Autodesk Fusion 360 part; units mm, degrees
(part 3 of 5)
sketch "Sketch16" plane through (0, 0, 0) normal (0, -1, 0) x (-1, 0, 0)
  arc A0 (122.6742, -5.0956) -> (122.6212, -5.0863) centre (122.616, -5.2713) ccw
  line L0 (123.102, -5.144) -> (123.0752, -5.1645)
  line L1 (124.5216, -5.1639) -> (123.8644, -5.1286)
  arc A1 (123.6043, -5.242) -> (123.5882, -5.1255) centre (123.5845, -5.1854) ccw
  arc A2 (123.8233, -5.6545) -> (123.7767, -5.422) centre (122.7524, -5.7482) ccw
  arc A3 (123.856, -5.4349) -> (123.9598, -5.5039) centre (123.9512, -5.4043) ccw
  line L2 (123.789, -5.2264) -> (123.856, -5.4349)
  line L3 (123.3395, -5.8789) -> (123.7146, -5.8461)
  line L4 (123.7767, -5.422) -> (123.7544, -5.352)
  line L5 (121.8655, -5.4934) -> (125.5172, -5.6276)
  line L6 (123.8282, -5.7107) -> (123.8233, -5.6545)
  spline S0 degree 5 poles (122.9975, -5.9023) (123.1042, -5.893) (123.156, -5.8823) (123.1472, -5.7594) (123.0188, -5.7281) (122.9135, -5.8224) (122.9975, -5.9023) knots 0 0 0 0 0 0 0.5 1 1 1 1 1 1
  line L7 (122.9975, -5.9023) -> (123.1042, -5.893) construction
  line L8 (123.1042, -5.893) -> (123.156, -5.8823) construction
  line L9 (123.156, -5.8823) -> (123.1472, -5.7594) construction
  line L10 (123.1472, -5.7594) -> (123.0188, -5.7281) construction
  line L11 (123.0188, -5.7281) -> (122.9135, -5.8224) construction
  line L12 (122.9135, -5.8224) -> (122.9975, -5.9023) construction
  arc A4 (123.0752, -5.1645) -> (123.1045, -5.339) centre (123.1359, -5.244) ccw
  arc A5 (123.7146, -5.8461) -> (123.8282, -5.7107) centre (123.7037, -5.7216) ccw
  line L13 (123.1447, -5.7836) -> (123.2791, -5.8649)
  spline S1 degree 5 poles (122.9292, -5.3527) (122.88, -5.3469) (122.8215, -5.3033) (122.8246, -5.224) (122.8952, -5.1732) (122.9827, -5.2223) (122.9881, -5.3313) (122.9292, -5.3527) knots 0 0 0 0 0 0 0.333333 0.666667 1 1 1 1 1 1
  line L14 (122.9292, -5.3527) -> (122.88, -5.3469) construction
  line L15 (122.88, -5.3469) -> (122.8215, -5.3033) construction
  line L16 (122.8215, -5.3033) -> (122.8246, -5.224) construction
  line L17 (122.8246, -5.224) -> (122.8952, -5.1732) construction
  line L18 (122.8952, -5.1732) -> (122.9827, -5.2223) construction
  line L19 (122.9827, -5.2223) -> (122.9881, -5.3313) construction
  line L20 (122.9881, -5.3313) -> (122.9292, -5.3527) construction
  arc A6 (122.3543, -5.2288) -> (122.4452, -5.3073) centre (122.4233, -5.2408) ccw
  spline S2 degree 5 poles (122.4306, -5.4713) (122.4226, -5.3565) (122.5709, -5.3131) (122.7774, -5.2403) (122.8192, -5.3704) (122.8155, -5.4904) (122.7473, -5.545) (122.638, -5.5931) (122.5038, -5.5663) (122.4306, -5.4713) knots 0 0 0 0 0 0 0.2 0.4 0.6 0.8 1 1 1 1 1 1
  line L21 (122.4306, -5.4713) -> (122.4226, -5.3565) construction
  line L22 (122.4226, -5.3565) -> (122.5709, -5.3131) construction
  line L23 (122.5709, -5.3131) -> (122.7774, -5.2403) construction
  line L24 (122.7774, -5.2403) -> (122.8192, -5.3704) construction
  line L25 (122.8192, -5.3704) -> (122.8155, -5.4904) construction
  line L26 (122.8155, -5.4904) -> (122.7473, -5.545) construction
  line L27 (122.7473, -5.545) -> (122.638, -5.5931) construction
  line L28 (122.638, -5.5931) -> (122.5038, -5.5663) construction
  line L29 (122.5038, -5.5663) -> (122.4306, -5.4713) construction
  line L30 (122.6144, -5.6431) -> (122.606, -5.6464)
  line L31 (122.5301, -5.7335) -> (122.5128, -5.8052)
  arc A7 (122.8103, -5.6413) -> (122.6144, -5.6431) centre (122.7147, -5.8992) ccw
  line L32 (123.6245, -5.2886) -> (123.351, -5.3896)
  line L33 (123.1045, -5.339) -> (123.1299, -5.3473)
  arc A8 (124.6146, -5.2458) -> (124.5216, -5.1639) centre (124.5163, -5.2637) ccw
  line L34 (124.861, -5.7338) -> (124.2595, -5.7864)
  line L35 (123.3066, -5.3458) -> (123.6043, -5.242)
  arc A9 (123.7544, -5.352) -> (123.6245, -5.2886) centre (123.6591, -5.3824) ccw
  line L36 (121.8838, -4.9975) -> (125.5316, -5.1315)
  arc A10 (123.8644, -5.1286) -> (123.789, -5.2264) centre (123.8604, -5.2035) ccw
  line L37 (123.5882, -5.1255) -> (123.2358, -5.1035)
  line L38 (125.5137, -5.7485) -> (121.8444, -6.0696)
  line L39 (123.9598, -5.5039) -> (124.5079, -5.4565)
  spline S3 degree 5 poles (123.9494, -5.8171) (123.8625, -5.7888) (123.8706, -5.5918) (123.9121, -5.5354) (124.1515, -5.4258) (124.1212, -5.8274) (123.9494, -5.8171) knots 0 0 0 0 0 0 0.5 1 1 1 1 1 1
  line L40 (123.9494, -5.8171) -> (123.8625, -5.7888) construction
  line L41 (123.8625, -5.7888) -> (123.8706, -5.5918) construction
  line L42 (123.8706, -5.5918) -> (123.9121, -5.5354) construction
  line L43 (123.9121, -5.5354) -> (124.1515, -5.4258) construction
  line L44 (124.1515, -5.4258) -> (124.1212, -5.8274) construction
  line L45 (124.1212, -5.8274) -> (123.9494, -5.8171) construction
  line L46 (122.6795, -5.0974) -> (122.6742, -5.0956)
  arc A11 (122.8042, -5.9191) -> (122.8961, -5.8717) centre (122.798, -5.7943) ccw
  line L47 (122.3617, -5.1862) -> (122.3543, -5.2288)
  arc A12 (122.5128, -5.8052) -> (122.615, -5.9286) centre (122.61, -5.8287) ccw
  arc A13 (122.9027, -5.8633) -> (122.9181, -5.7333) centre (122.8047, -5.7858) ccw
  arc A14 (122.606, -5.6464) -> (122.5301, -5.7335) centre (122.6516, -5.7628) ccw
  spline S4 degree 5 poles (122.0426, -5.9763) (121.8729, -5.8903) (122.0398, -5.5137) (122.2556, -5.9869) (122.144, -6.0042) (122.0426, -5.9763) knots 0 0 0 0 0 0 1 1 1 1 1 1
  line L48 (122.0426, -5.9763) -> (121.8729, -5.8903) construction
  line L49 (121.8729, -5.8903) -> (122.0398, -5.5137) construction
  line L50 (122.0398, -5.5137) -> (122.2556, -5.9869) construction
  line L51 (122.2556, -5.9869) -> (122.144, -6.0042) construction
  line L52 (122.144, -6.0042) -> (122.0426, -5.9763) construction
  line L53 (122.8961, -5.8717) -> (122.9027, -5.8633)
  line L54 (122.615, -5.9286) -> (122.8042, -5.9191)
  line L55 (122.4452, -5.3073) -> (122.6793, -5.2304)
  arc A15 (122.9194, -5.7361) -> (122.8213, -5.6454) centre (122.7605, -5.8095) ccw
  line L56 (122.6212, -5.0863) -> (122.4884, -5.0826)
  line L57 (124.7695, -5.5577) -> (124.8858, -5.6544)
  line L58 (124.6105, -5.223) -> (124.6146, -5.2458)
  arc A16 (125.0173, -5.6732) -> (125.1878, -5.7213) centre (125.166, -5.4723) ccw
  line L59 (124.8259, -5.5315) -> (125.0173, -5.6732)
  spline S5 degree 5 poles (123.0947, -5.5531) (123.1905, -5.4657) (123.1798, -5.3896) (123.0478, -5.3646) (122.9193, -5.4022) (122.7897, -5.5433) (122.8659, -5.6259) (122.9658, -5.6557) (123.0537, -5.6399) (123.0947, -5.5531) knots 0 0 0 0 0 0 0.2 0.4 0.6 0.8 1 1 1 1 1 1
  line L60 (123.0947, -5.5531) -> (123.1905, -5.4657) construction
  line L61 (123.1905, -5.4657) -> (123.1798, -5.3896) construction
  line L62 (123.1798, -5.3896) -> (123.0478, -5.3646) construction
  line L63 (123.0478, -5.3646) -> (122.9193, -5.4022) construction
  line L64 (122.9193, -5.4022) -> (122.7897, -5.5433) construction
  line L65 (122.7897, -5.5433) -> (122.8659, -5.6259) construction
  line L66 (122.8659, -5.6259) -> (122.9658, -5.6557) construction
  line L67 (122.9658, -5.6557) -> (123.0537, -5.6399) construction
  line L68 (123.0537, -5.6399) -> (123.0947, -5.5531) construction
  arc A17 (125.4261, -5.2886) -> (125.3296, -5.1836) centre (125.3262, -5.2835) ccw
  arc A18 (123.116, -5.6386) -> (123.1447, -5.7836) centre (123.1964, -5.6981) ccw
  line L69 (125.3296, -5.1836) -> (124.7854, -5.1648)
  line L70 (123.2366, -5.4755) -> (123.116, -5.6386)
  arc A19 (124.861, -5.7338) -> (124.8858, -5.6544) centre (124.8571, -5.689) ccw
  arc A20 (123.351, -5.3896) -> (123.2366, -5.4755) centre (123.4377, -5.6241) ccw
  arc A21 (124.1566, -5.7201) -> (124.2595, -5.7864) centre (124.2508, -5.6868) ccw
  arc A22 (123.2791, -5.8649) -> (123.3395, -5.8789) centre (123.3308, -5.7793) ccw
  line L71 (124.1498, -5.6486) -> (124.1499, -5.6497)
  arc A23 (123.2358, -5.1035) -> (123.102, -5.144) centre (123.2233, -5.3031) ccw
  line L72 (125.5316, -5.1315) -> (125.5137, -5.7485)
  arc A24 (124.2379, -5.5417) -> (124.1499, -5.6497) centre (124.2495, -5.641) ccw
  line L73 (125.4094, -5.6154) -> (125.4261, -5.2886)
  arc A25 (123.1299, -5.3473) -> (123.3066, -5.3458) centre (123.2161, -5.0862) ccw
  line L74 (125.1878, -5.7213) -> (125.3183, -5.7099)
  arc A26 (125.3183, -5.7099) -> (125.4094, -5.6154) centre (125.3096, -5.6103) ccw
  line L75 (124.1566, -5.7201) -> (124.1559, -5.7183)
  arc A27 (124.6914, -5.3208) -> (124.8259, -5.5315) centre (125.0342, -5.2502) ccw
  line L76 (124.2379, -5.5417) -> (124.5806, -5.5016)
  line L77 (124.684, -5.2849) -> (124.6914, -5.3208)
  arc A28 (124.7854, -5.1648) -> (124.684, -5.2849) centre (124.7819, -5.2647) ccw
  arc A29 (124.7695, -5.5577) -> (124.5806, -5.5016) centre (124.6097, -5.7499) ccw
  line L78 (124.6271, -5.3138) -> (124.6105, -5.223)
  line L79 (124.1559, -5.7183) -> (124.1498, -5.6486)
  arc A30 (124.5079, -5.4565) -> (124.6136, -5.3988) centre (124.495, -5.3071) ccw
  arc A31 (124.6136, -5.3988) -> (124.6271, -5.3138) centre (124.4992, -5.3372) ccw
  line L80 (122.8213, -5.6454) -> (122.8103, -5.6413)
  line L81 (121.8444, -6.0696) -> (121.8838, -4.9975)
  spline S6 degree 5 poles (122.2381, -5.4004) (122.0382, -5.4442) (121.8814, -5.4184) (122.1972, -5.96) (122.3884, -6.05) (122.4454, -5.8928) (122.5168, -5.7223) (122.3409, -5.3698) (122.2381, -5.4004) knots 0 0 0 0 0 0 0.25 0.5 0.75 1 1 1 1 1 1
  line L82 (122.2381, -5.4004) -> (122.0382, -5.4442) construction
  line L83 (122.0382, -5.4442) -> (121.8814, -5.4184) construction
  line L84 (121.8814, -5.4184) -> (122.1972, -5.96) construction
  line L85 (122.1972, -5.96) -> (122.3884, -6.05) construction
  line L86 (122.3884, -6.05) -> (122.4454, -5.8928) construction
  line L87 (122.4454, -5.8928) -> (122.5168, -5.7223) construction
  line L88 (122.5168, -5.7223) -> (122.3409, -5.3698) construction
  line L89 (122.3409, -5.3698) -> (122.2381, -5.4004) construction
  arc A32 (122.6793, -5.2304) -> (122.6795, -5.0974) centre (122.6575, -5.1639) ccw
  arc A33 (122.1383, -5.3484) -> (122.2847, -5.1559) centre (122.0847, -5.1557) ccw
  line L90 (122.2098, -5.0785) -> (122.1123, -5.0784)
  line L91 (122.0124, -5.1715) -> (122.0048, -5.2817)
  line L92 (122.2847, -5.1559) -> (122.2847, -5.1536)
  arc A34 (122.4884, -5.0826) -> (122.3617, -5.1862) centre (122.4849, -5.2076) ccw
  arc A35 (122.0048, -5.2817) -> (122.0998, -5.3591) centre (122.0797, -5.2869) ccw
  arc A36 (122.2847, -5.1536) -> (122.2098, -5.0785) centre (122.2097, -5.1535) ccw
  arc A37 (122.1123, -5.0784) -> (122.0124, -5.1715) centre (122.1122, -5.1784) ccw
  line L93 (122.9181, -5.7333) -> (122.9194, -5.7361)
  line L94 (122.0998, -5.3591) -> (122.1383, -5.3484)
  arc A38 (101.6624, -9.2829) -> (105.8159, -15.1808) centre (107.6246, -9.4955) ccw
  arc A39 (70.9904, -13.8268) -> (76.2587, -14.0644) centre (73.9745, -6.1856) ccw
  arc A40 (89.9571, -7.1067) -> (89.8164, -11.0703) centre (90.5403, -9.1117) ccw
  line L95 (91.7075, -6.8404) -> (95.6704, -6.8748)
  arc A41 (109.7609, -10.0454) -> (106.8858, -7.1606) centre (106.7795, -10.1417) ccw
  arc A42 (99.3328, -10.1021) -> (95.6704, -6.8748) centre (95.6379, -10.6034) ccw
  line L96 (43.0155, -18.6474) -> (32.8431, -17.0766)
  line L97 (45.2455, -24.0556) -> (45.2666, -24.0022)
  line L98 (34.971, -7.0748) -> (54.6013, -6.7408)
  arc A43 (106.9529, -15.5425) -> (109.8673, -13.3383) centre (107.6312, -13.4105) ccw
  line L99 (45.5246, -21.9308) -> (45.5205, -21.9641)
  spline S7 degree 5 poles (96.9668, -18.5257) (97.3315, -15.1102) (92.9589, -13.6548) (86.882, -11.2585) (85.4937, -15.0929) (85.4728, -18.6727) (87.4465, -20.3757) (90.6533, -21.9288) (94.6811, -21.2769) (96.9668, -18.5257) knots 0 0 0 0 0 0 0.2 0.4 0.6 0.8 1 1 1 1 1 1
  line L100 (96.9668, -18.5257) -> (97.3315, -15.1102) construction
  line L101 (97.3315, -15.1102) -> (92.9589, -13.6548) construction
  line L102 (92.9589, -13.6548) -> (86.882, -11.2585) construction
  line L103 (86.882, -11.2585) -> (85.4937, -15.0929) construction
  line L104 (85.4937, -15.0929) -> (85.4728, -18.6727) construction
  line L105 (85.4728, -18.6727) -> (87.4465, -20.3757) construction
  line L106 (87.4465, -20.3757) -> (90.6533, -21.9288) construction
  line L107 (90.6533, -21.9288) -> (94.6811, -21.2769) construction
  line L108 (94.6811, -21.2769) -> (96.9668, -18.5257) construction
  line L109 (90.9724, -31.9544) -> (85.3412, -31.4649)
  line L110 (109.7609, -10.0454) -> (109.8673, -13.3383)
  line L111 (55.0443, -24.1326) -> (55.2523, -22.4622)
  arc A44 (91.3008, -23.4448) -> (85.4647, -23.1768) centre (88.0311, -30.9683) ccw
  arc A45 (56.7428, -9.7399) -> (54.6013, -6.7408) centre (54.6394, -8.9777) ccw
  arc A46 (91.7075, -6.8404) -> (90.1182, -7.0598) centre (91.6595, -12.3587) ccw
  line L112 (106.9529, -15.5425) -> (105.8159, -15.1808)
  line L113 (96.7132, -13.6191) -> (89.8164, -11.0703)
  spline S8 degree 5 poles (51.3155, -27.1729) (53.937, -26.4249) (53.9111, -20.5433) (52.7356, -18.8166) (45.7166, -15.2876) (46.1809, -27.2918) (51.3155, -27.1729) knots 0 0 0 0 0 0 0.5 1 1 1 1 1 1
  line L114 (51.3155, -27.1729) -> (53.937, -26.4249) construction
  line L115 (53.937, -26.4249) -> (53.9111, -20.5433) construction
  line L116 (53.9111, -20.5433) -> (52.7356, -18.8166) construction
  line L117 (52.7356, -18.8166) -> (45.7166, -15.2876) construction
  line L118 (45.7166, -15.2876) -> (46.1809, -27.2918) construction
  line L119 (46.1809, -27.2918) -> (51.3155, -27.1729) construction
  line L120 (101.6624, -9.2829) -> (101.6649, -9.2131)
  arc A47 (56.8948, -15.5841) -> (55.2523, -22.4622) centre (87.0737, -26.4258) ccw
  line L121 (69.427, -29.6816) -> (58.2835, -28.2936)
  line L122 (89.9571, -7.1067) -> (90.1182, -7.0598)
  arc A48 (55.0443, -24.1326) -> (58.2835, -28.2936) centre (58.7444, -24.5935) ccw
  arc A49 (96.7132, -13.6191) -> (99.5062, -11.3798) centre (97.4371, -11.6605) ccw
  line L123 (103.9805, -7.057) -> (106.8858, -7.1606)
  line L124 (99.3328, -10.1021) -> (99.5062, -11.3798)
  line L125 (75.3395, -27.0549) -> (71.244, -29.3293)
  arc A50 (62.837, -6.95) -> (62.232, -10.4064) centre (62.8831, -8.7392) ccw
  arc A51 (42.1027, -25.919) -> (45.2455, -24.0556) centre (42.4714, -22.9589) ccw
  line L126 (51.3477, -17.8246) -> (35.0606, -15.8132)
  arc A52 (103.9805, -7.057) -> (101.6649, -9.2131) centre (103.9007, -9.2928) ccw
  line L127 (113.7873, -4.9975) -> (4.8993, -5.006)
  arc A53 (72.9355, -17.7672) -> (69.6198, -15.0822) centre (66.7806, -21.9782) ccw
  line L128 (4.7576, -23.4188) -> (113.7898, -36.9995)
  line L129 (113.7884, -19.7997) -> (4.7873, -13.6679)
  line L130 (62.837, -6.95) -> (73.3676, -6.6788)
  line L131 (61.5787, -11.7716) -> (69.6198, -15.0822)
  line L132 (4.8993, -5.006) -> (4.7576, -23.4188)
  arc A54 (25.4984, -17.7008) -> (29.7394, -11.5664) centre (19.5973, -9.0879) ccw
  arc A55 (32.8431, -17.0766) -> (27.15, -18.542) centre (31.7051, -24.4468) ccw
  line L133 (32.258, -8.7389) -> (32.1089, -9.414)
  arc A56 (8.012, -19.5628) -> (10.626, -22.4806) centre (10.9947, -19.5204) ccw
  line L134 (25.4984, -17.7008) -> (19.6392, -21.7151)
  arc A57 (14.5024, -22.9634) -> (19.6392, -21.7151) centre (15.4242, -15.5631) ccw
  line L135 (56.8948, -15.5841) -> (57.6358, -13.5215)
  line L136 (14.5024, -22.9634) -> (10.626, -22.4806)
  line L137 (70.9904, -13.8268) -> (62.232, -10.4064)
  line L138 (24.2313, -23.693) -> (42.1027, -25.919)
  arc A58 (29.9989, -10.5044) -> (27.1075, -6.8132) centre (27.1011, -9.7962) ccw
  arc A59 (10.8624, -6.7785) -> (7.8733, -9.8039) centre (10.856, -9.7615) ccw
  line L139 (27.15, -18.542) -> (23.5773, -21.2981)
  arc A60 (31.6639, -11.4287) -> (31.9714, -13.9779) centre (35.4505, -12.2651) ccw
  line L140 (91.3008, -23.4448) -> (91.548, -23.5522)
  arc A61 (31.9714, -13.9779) -> (35.0606, -15.8132) centre (35.609, -11.3724) ccw
  arc A62 (23.5773, -21.2981) -> (24.2313, -23.693) centre (24.3972, -22.361) ccw
  line L141 (10.8624, -6.7785) -> (27.1075, -6.8132)
  line L142 (8.012, -19.5628) -> (7.8733, -9.8039)
  arc A63 (34.971, -7.0748) -> (32.1089, -9.414) centre (35.0217, -10.0574) ccw
  line L143 (72.9355, -17.7672) -> (76.3532, -22.7627)
  line L144 (31.6639, -11.4287) -> (32.258, -8.7389)
  line L145 (113.7898, -36.9995) -> (113.7873, -4.9975)
  line L146 (45.2666, -24.0022) -> (45.5246, -21.9308)
  line L147 (29.9989, -10.5044) -> (29.7394, -11.5664)
  line L148 (56.7428, -9.7399) -> (54.5179, -15.8803)
  spline S9 degree 5 poles (107.9837, -34.0023) (113.1348, -31.6237) (108.5717, -20.2166) (101.6226, -34.085) (104.9302, -34.7228) (107.9837, -34.0023) knots 0 0 0 0 0 0 1 1 1 1 1 1
  line L149 (107.9837, -34.0023) -> (113.1348, -31.6237) construction
  line L150 (113.1348, -31.6237) -> (108.5717, -20.2166) construction
  line L151 (108.5717, -20.2166) -> (101.6226, -34.085) construction
  line L152 (101.6226, -34.085) -> (104.9302, -34.7228) construction
  line L153 (104.9302, -34.7228) -> (107.9837, -34.0023) construction
  spline S10 degree 5 poles (77.0809, -20.2383) (74.3221, -17.5267) (74.7247, -15.2695) (78.6853, -14.6699) (82.4748, -15.9313) (86.1835, -20.2791) (83.823, -22.6567) (80.8115, -23.4352) (78.2106, -22.8684) (77.0809, -20.2383) knots 0 0 0 0 0 0 0.2 0.4 0.6 0.8 1 1 1 1 1 1
  line L154 (77.0809, -20.2383) -> (74.3221, -17.5267) construction
  line L155 (74.3221, -17.5267) -> (74.7247, -15.2695) construction
  line L156 (74.7247, -15.2695) -> (78.6853, -14.6699) construction
  line L157 (78.6853, -14.6699) -> (82.4748, -15.9313) construction
  line L158 (82.4748, -15.9313) -> (86.1835, -20.2791) construction
  line L159 (86.1835, -20.2791) -> (83.823, -22.6567) construction
  line L160 (83.823, -22.6567) -> (80.8115, -23.4352) construction
  line L161 (80.8115, -23.4352) -> (78.2106, -22.8684) construction
  line L162 (78.2106, -22.8684) -> (77.0809, -20.2383) construction
  spline S11 degree 5 poles (102.7832, -16.62) (108.6944, -18.1458) (113.3986, -17.5474) (103.3913, -33.3483) (97.5924, -35.8202) (96.0663, -31.0721) (94.1248, -25.9135) (99.7525, -15.5964) (102.7832, -16.62) knots 0 0 0 0 0 0 0.25 0.5 0.75 1 1 1 1 1 1
  line L163 (102.7832, -16.62) -> (108.6944, -18.1458) construction
  line L164 (108.6944, -18.1458) -> (113.3986, -17.5474) construction
  line L165 (113.3986, -17.5474) -> (103.3913, -33.3483) construction
  line L166 (103.3913, -33.3483) -> (97.5924, -35.8202) construction
  line L167 (97.5924, -35.8202) -> (96.0663, -31.0721) construction
  line L168 (96.0663, -31.0721) -> (94.1248, -25.9135) construction
  line L169 (94.1248, -25.9135) -> (99.7525, -15.5964) construction
  line L170 (99.7525, -15.5964) -> (102.7832, -16.62) construction
  arc A64 (77.31, -8.0343) -> (73.3676, -6.6788) centre (73.5212, -12.6428) ccw
  arc A65 (61.5787, -11.7716) -> (57.6358, -13.5215) centre (60.4431, -14.53) ccw
  arc A66 (45.5205, -21.9641) -> (43.0155, -18.6474) centre (42.5603, -21.5954) ccw
  line L171 (77.0236, -13.8427) -> (76.2587, -14.0644)
  line L172 (85.13, -23.287) -> (85.4647, -23.1768)
  spline S12 degree 5 poles (82.235, -14.4442) (83.7072, -14.324) (85.5003, -13.0901) (85.4918, -10.721) (83.4434, -9.1301) (80.7835, -10.4989) (80.5009, -13.7424) (82.235, -14.4442) knots 0 0 0 0 0 0 0.333333 0.666667 1 1 1 1 1 1
  line L173 (82.235, -14.4442) -> (83.7072, -14.324) construction
  line L174 (83.7072, -14.324) -> (85.5003, -13.0901) construction
  line L175 (85.5003, -13.0901) -> (85.4918, -10.721) construction
  line L176 (85.4918, -10.721) -> (83.4434, -9.1301) construction
  line L177 (83.4434, -9.1301) -> (80.7835, -10.4989) construction
  line L178 (80.7835, -10.4989) -> (80.5009, -13.7424) construction
  line L179 (80.5009, -13.7424) -> (82.235, -14.4442) construction
  line L180 (77.31, -8.0343) -> (78.0873, -8.6734)
  arc A67 (90.9724, -31.9544) -> (94.1541, -28.3895) centre (91.2307, -28.9826) ccw
  spline S13 degree 5 poles (79.5966, -30.7522) (76.4277, -30.3575) (74.8955, -29.9845) (75.29, -26.3298) (79.1534, -25.536) (82.1888, -28.4642) (79.5966, -30.7522) knots 0 0 0 0 0 0 0.5 1 1 1 1 1 1
  line L181 (79.5966, -30.7522) -> (76.4277, -30.3575) construction
  line L182 (76.4277, -30.3575) -> (74.8955, -29.9845) construction
  line L183 (74.8955, -29.9845) -> (75.29, -26.3298) construction
  line L184 (75.29, -26.3298) -> (79.1534, -25.536) construction
  line L185 (79.1534, -25.536) -> (82.1888, -28.4642) construction
  line L186 (82.1888, -28.4642) -> (79.5966, -30.7522) construction
  arc A68 (82.149, -25.8024) -> (82.4648, -29.6924) centre (85.4739, -27.4902) ccw
  arc A69 (82.6551, -29.9524) -> (85.3412, -31.4649) centre (85.6641, -27.7502) ccw
  line L187 (93.7161, -26.2305) -> (94.1541, -28.3895)
  arc A70 (77.0236, -13.8427) -> (78.0873, -8.6734) centre (76.1929, -10.9777) ccw
  arc A71 (51.3477, -17.8246) -> (54.5179, -15.8803) centre (51.7133, -14.8641) ccw
  line L188 (82.149, -25.8024) -> (82.1084, -25.8823)
  arc A72 (85.13, -23.287) -> (82.1084, -25.8823) centre (86.7632, -28.2452) ccw
  arc A73 (93.7161, -26.2305) -> (91.548, -23.5522) centre (90.0618, -26.972) ccw
  line L189 (82.6551, -29.9524) -> (82.4648, -29.6924)
  arc A74 (75.3395, -27.0549) -> (76.3532, -22.7627) centre (73.8913, -24.447) ccw
  arc A75 (69.427, -29.6816) -> (71.244, -29.3293) centre (69.7957, -26.7215) ccw
  line L190 (113.7873, -37.3) -> (113.7873, -4.9975)
  line L191 (113.7873, -4.9975) -> (4.7873, -4.9975)
  line L192 (4.7873, -4.9975) -> (4.7873, -23.5975)
  line L193 (4.7873, -23.5975) -> (113.7873, -37.3)
  point P0 (113.7873, -4.9975)
  dimension "d385" = 0.07
  dimension "d386" = 0.07
  dimension "d387" = 0.185
  dimension "d388" = 0.125
  dimension "d389" = 0.1
  dimension "d390" = 0.275
  dimension "d391" = 0.2
  dimension "d392" = 0.06
  dimension "d393" = 0.1
  dimension "d394" = 0.35
  dimension "d395" = 0.25
  dimension "d396" = 0.1
  dimension "d397" = 0.1
  dimension "d398" = 0.1
  dimension "d399" = 0.1
  dimension "d400" = 0.25
  dimension "d401" = 0.045
  dimension "d402" = 0.13
  dimension "d403" = 0.1
  dimension "d404" = 0.075
  dimension "d405" = 0.1
  dimension "d406" = 0.25
  dimension "d407" = 0.1
  dimension "d408" = 1.075
  dimension "d409" = 0.125
  dimension "d410" = 0.1
  dimension "d411" = 0.125
  dimension "d412" = 0.125
  dimension "d413" = 0.175
  dimension "d414" = 0.275
  dimension "d415" = 0.125
  dimension "d416" = 0.075
  dimension "d417" = 0.1
  dimension "d418" = 0.075
  dimension "d419" = 0.2
  constraint perpendicular L36 L81
  constraint coincident S4.start S4.end
  constraint coincident S6.start S6.end
  constraint tangent A6 L47
  constraint tangent A6 L55
  constraint tangent L55 A32
  constraint tangent L46 A32
  constraint tangent A0 L46
  constraint tangent A0 L56
  constraint tangent L56 A34
  constraint tangent L47 A34
  constraint tangent L0 A4
  constraint tangent A4 L33
  constraint tangent L35 A25
  constraint tangent L33 A25
  constraint tangent L37 A23
  constraint tangent L0 A23
  constraint tangent A1 L35
  constraint tangent A1 L37
  constraint parallel L38 L74
  constraint tangent L69 A28
  constraint tangent L77 A28
  constraint tangent A27 L77
  constraint tangent L59 A27
  constraint tangent A16 L59
  constraint tangent A16 L74
  constraint tangent A17 L69
  constraint tangent A17 L73
  constraint tangent L74 A26
  constraint tangent L73 A26
  constraint parallel L71 L79
  constraint tangent L34 A21
  constraint tangent A21 L75
  constraint tangent A24 L76
  constraint tangent L71 A24
  constraint tangent L76 A29
  constraint tangent L57 A29
  constraint tangent L57 A19
  constraint tangent L34 A19
  constraint parallel L58 L78
  constraint tangent L39 A30
  constraint tangent L78 A31
  constraint coincident A30.end A31.start
  constraint tangent A3 L39
  constraint tangent A3 L2
  constraint tangent A8 L58
  constraint tangent L1 A8
  constraint equal A3 A8
  constraint tangent L1 A10
  constraint tangent L2 A10
  constraint coincident S3.start S3.end
  constraint parallel L3 L38
  constraint perpendicular L6 L38
  constraint tangent L3 A22
  constraint tangent L13 A22
  constraint tangent A18 L70
  constraint tangent L13 A18
  constraint equal A18 A22
  constraint tangent L32 A20
  constraint tangent L70 A20
  constraint tangent L4 A9
  constraint tangent L32 A9
  constraint tangent A2 L6
  constraint tangent A2 L4
  constraint tangent L3 A5
  constraint tangent L6 A5
  constraint coincident S0.start S0.end
  constraint coincident S1.start S1.end
  constraint coincident S5.start S5.end
  constraint coincident S2.start S2.end
  constraint tangent A12 L54
  constraint tangent L31 A12
  constraint tangent A11 L54
  constraint tangent A11 L53
  constraint tangent A13 L53
  constraint tangent A13 L93
  constraint tangent A15 L93
  constraint tangent A15 L80
  constraint tangent A7 L80
  constraint tangent L30 A7
  constraint tangent L30 A14
  constraint tangent L31 A14
  constraint perpendicular L90 L92
  constraint tangent A35 L94
  constraint tangent L91 A35
  constraint tangent L90 A37
  constraint tangent L91 A37
  constraint tangent L92 A36
  constraint tangent L90 A36
  constraint tangent A33 L94
  constraint tangent A33 L92
  constraint coincident L5.start L81
  constraint coincident L5.end L72
  constraint perpendicular L5 L81
  constraint coincident L129.end L192
  measures "d385" radius of A6
  measures "d386" radius of A32
  measures "d387" radius of A0
  measures "d388" radius of A34
  measures "d389" radius of A4
  measures "d390" radius of A25
  measures "d391" radius of A23
  measures "d392" radius of A1
  measures "d393" radius of A28
  measures "d394" radius of A27
  measures "d395" radius of A16
  measures "d396" radius of A17
  measures "d397" radius of A26
  measures "d398" radius of A21
  measures "d399" radius of A24
  measures "d400" radius of A29
  measures "d401" radius of A19
  measures "d402" radius of A31
  measures "d403" radius of A3
  measures "d404" radius of A10
  measures "d405" radius of A22
  measures "d406" radius of A20
  measures "d407" radius of A9
  measures "d408" radius of A2
  measures "d409" radius of A5
  measures "d410" radius of A12
  measures "d411" radius of A11
  measures "d412" radius of A13
  measures "d413" radius of A15
  measures "d414" radius of A7
  measures "d415" radius of A14
  measures "d416" radius of A35
  measures "d417" radius of A37
  measures "d418" radius of A36
  measures "d419" radius of A33
sketch "Sketch17" plane through (-59.2873, 0, 21.1488) normal (0, -1, 0) x (1, 0, 0)
  line L0 (-54.5012, -1.3491) -> (54.5, -7.4809)
sketch "Sketch18" plane through (-4.7873, 0, 0) normal (1, 0, 0) x (0, 1, 0)
  line L0 (0, 23.5975) -> (0, 4.9975)
  line L1 (0, 4.9975) -> (300, 4.9975)
  line L2 (300, 4.9975) -> (300, 23.5975)
  line L3 (300, 23.5975) -> (0, 23.5975)
  line L4 (300, 37.3) -> (0, 37.3)
  line L5 (1.4675, 37.3) -> (298.5325, 37.3)
  line L6 (1.4675, 37.3) -> (0, 13.6679)
  line L7 (0, 13.6679) -> (0, 37.3)
  line L8 (1.4675, 37.3) -> (0, 37.3)
  line L9 (1.4675, 37.3) -> (1.4675, 4.9975)
  line L10 (1.4675, 4.9975) -> (0, 4.9975)
  line L11 (0, 13.6679) -> (1.4675, 4.9975)
  line L12 (0, 13.6679) -> (0, 4.9975)
  point P0 (1.4675, 23.5971)
  point P1 (0, 13.6679)
  constraint coincident L5.start L6.start
  constraint coincident P1 L6.end
  constraint coincident L4.end L7.end
  constraint coincident L1 L9.end
  constraint perpendicular L1 L9
  constraint coincident L0.end L1.start
ref_plane "WorkPlane5" through (-4.7873, 150, 4.9975) normal (0.992546, 0, -0.121869) x (0, 1, 0)
sketch "Sketch19" plane through (-5.3207, 0, 0.6533) normal (0.992546, 0, -0.121869) x (0, 1, 0)
  line L0 (0, 4.3768) -> (300, 4.3768)
  line L1 (1.4675, 36.4386) -> (0, 36.4386)
  line L2 (0, -8.907) -> (1.4675, -8.907)
  line L3 (1.4675, 36.4386) -> (0, 36.4386)
  line L4 (1.4675, 36.4386) -> (1.4675, -8.907)
  line L5 (1.4675, 36.4386) -> (0, 36.4386)
  line L6 (2, 6.9859) -> (1.4675, -8.907)
  line L7 (2, 6.9859) -> (1.4675, 36.4386)
  line L8 (0, 4.3768) -> (300, 4.3768)
  line L9 (150, -19.0201) -> (150, -52.6146)
  line L10 (298.5325, 36.4386) -> (298.5325, -8.907)
  line L11 (298, 6.9859) -> (298.5325, 36.4386)
  line L12 (298.5325, 36.4386) -> (304, 36.4386)
  line L13 (299.3952, 36.6527) -> (298, 6.9859)
  line L14 (298, 6.9859) -> (298.5325, -8.907)
  line L15 (298, 6.9859) -> (299.2437, -9.2706)
  line L16 (304, -8.907) -> (298.5325, -8.907)
  line L17 (2, 36.4386) -> (2, -8.907)
  line L18 (-3.864, 36.4386) -> (0, 36.4386)
  line L19 (0, 36.4386) -> (0, -8.907)
  line L20 (0, -8.907) -> (-3.864, -8.907)
  line L21 (-3.864, -8.907) -> (-3.864, 36.4386)
  line L22 (304, 36.4386) -> (314.0835, 36.4386)
  line L23 (314.0835, 36.4386) -> (314.0835, -8.907)
  line L24 (314.0835, -8.907) -> (304, -8.907)
  line L25 (304, -8.907) -> (304, 36.4386)
  point P0 (0, 12.9826)
  point P1 (0, -8.907)
  dimension "d428" = 300
  dimension "d429" = 150
  dimension "d658" = 2
  constraint coincident P1 L2.start
  constraint horizontal L2
  constraint coincident L1.start L3.start
  constraint coincident L1.end L3.end
  constraint perpendicular L2 L4
  constraint vertical L9
  constraint symmetric L1.start L9 L10.start
  constraint symmetric L2.end L9 L10.end
  constraint symmetric L6.start L9 L11.start
  constraint coincident L5 L17.start
  constraint coincident L2 L17.end
  constraint perpendicular L2 L17
  constraint coincident L6.start L17
  constraint horizontal L18
  constraint vertical L19
  constraint horizontal L20
  constraint vertical L21
  constraint horizontal L22
  constraint vertical L23
  constraint horizontal L24
  constraint vertical L25
  measures "d428" distance of L0.start L0.end
  measures "d429" distance of L0.end L9
  measures "d658" distance of L17 L19
extrude "Extrude5" cut sketch "Sketch19" against normal through all contours L0 L1 L3 L4 L5 L8 L19 | L18 L19 L20 L21 | L0 L2 L4 L8 L19 | L0 L4 L6 L7 L8 | L0 L4 L6 L8
ref_plane "WorkPlane6" through (-60.9169, 5.1376, 13.5198) normal (0, 1, 0) x (-0.992191, 0, 0.12473)
extrude "Extrude6" cut sketch "Sketch16" against normal up to surface (5.1376 mm away) contours A38 A41 A43 L110 L112 L120 L123 A52 | A39 A50 L130 L137 A64 L171 L180 A70 | A40 L95 A42 A46 L113 L122 A49 L124 | L96 L97 L99 A51 A55 L138 L139 A62 L146 A66 | L98 A45 L129 A60 A61 A63 L144 L148 A71 | L126 L129 A61 A71 | L111 A47 L121 A48 L125 A53 L129 L143 A74 A75 | A47 A53 L129 L131 L135 A65 | L129 A54 A56 L134 A57 L136 L142 | L129 A54 A58 A59 L141 L142 L147 | L129 S10 | L129 S10 | S7 L129 | S7 L129 | L129 S11 | L129 S11 | L109 A44 L140 L172 A67 A68 A69 L187 L188 A72 A73 L189 | S8 | S9 | S12 | S13
extrude "Extrude7" cut sketch "Sketch16" against normal up to surface (5.1376 mm away) contours A39 A50 L130 L137 A64 L171 L180 A70 | L96 L97 L99 A51 A55 L138 L139 A62 L146 A66 | L98 A45 L129 A60 A61 A63 L144 L148 A71 | L126 L129 A61 A71 | L111 A47 L121 A48 L125 A53 L129 L143 A74 A75 | A47 A53 L129 L131 L135 A65 | L129 S10 | L129 S10 | S7 L129 | S7 L129 | L109 A44 L140 L172 A67 A68 A69 L187 L188 A72 A73 L189 | S8 | S13
chamfer "Chamfer1" distance 1.25 angle 45 6 edges at (-4.7873, 1.8567, 15.6118) (-4.7873, 1.9563, 6.3118) (-59.2873, 1.69, 4.9975) (-59.2873, 1.7105, 30.4488) (-113.7873, 1.8538, 29.1549) (-113.7873, 1.7338, 13.0036)
extrude "Extrude8" cut sketch "Sketch19" against normal through all contours L0 L8 L14 L15 | L0 L8 L10 L14 L15 | L0 L8 L10 L13 L15 | L0 L8 L10 L15 | L10 L11 L13 | L10 L15 L16 | L10 L12 L13 L15 L16 L25 | L10 L12 L13 | L22 L23 L24 L25
ref_plane "WorkPlane7" through (-9.6857, 150, -34.8971) normal (0, 1, 0) x (-0.121869, 0, -0.992546)
ref_plane "WorkPlane8" through (-59.2857, 298.5325, 30.4486) normal (0, 1, 0) x (0.992191, 0, -0.12473)
mirror "Mirror1" about plane through (-9.6857, 150, -34.8971) normal (0, 1, 0) of "Extrude7"
mirror "Mirror2" about plane through (-9.6857, 150, -34.8971) normal (0, 1, 0) of "Extrude6"
ref_plane "WorkPlane9" through (-105.2128, 298, 19.9569) normal (0, 1, 0) x (0.992546, 0, -0.121869)
sketch "Sketch20" plane through (0, 298, 0) normal (0, 1, 0) x (1, 0, 0)
  spline S0 degree 5 poles (-102.7832, -16.62) (-108.6944, -18.1458) (-113.3986, -17.5474) (-103.3913, -33.3483) (-97.5924, -35.8202) (-96.0663, -31.0721) (-94.1248, -25.9135) (-99.7525, -15.5964) (-102.7832, -16.62) knots 0 0 0 0 0 0 0.25 0.5 0.75 1 1 1 1 1 1
extrude "Extrude9" cut sketch "Sketch20" along normal up to surface (0.5325 mm away)
sketch "Sketch22" plane through (-4.7873, 0, 0) normal (1, 0, 0) x (0, 1, 0)
  line L0 (298, 7.6262) -> (298.2866, 23.5975)
  line L1 (298.2866, 23.5975) -> (2.9636, 23.5975)
  line L2 (3.1633, 4.9975) -> (298.0874, 4.9975)
  line L3 (298.0874, 4.9975) -> (298, 7.6262)
  line L4 (10.4246, 20.4636) -> (4.1693, 11.2495)
  line L5 (5.8136, 8.1262) -> (12.4356, 8.0915)
  line L6 (14.9486, 10.5784) -> (14.993, 19.0463)
  arc A0 (14.993, 19.0463) -> (10.4246, 20.4636) centre (12.493, 19.0594) ccw
  arc A1 (12.4356, 8.0915) -> (14.9486, 10.5784) centre (12.4487, 10.5915) ccw
  arc A2 (4.1693, 11.2495) -> (5.8136, 8.1262) centre (5.824, 10.1262) ccw
  line L7 (17.9622, 17.2008) -> (17.9226, 9.6257)
  line L8 (19.4147, 8.1178) -> (25.6764, 8.085)
  line L9 (26.8453, 10.5346) -> (20.6233, 18.1425)
  arc A3 (20.6233, 18.1425) -> (17.9622, 17.2008) centre (19.4622, 17.1929) ccw
  arc A4 (17.9226, 9.6257) -> (19.4147, 8.1178) centre (19.4225, 9.6178) ccw
  arc A5 (25.6764, 8.085) -> (26.8453, 10.5346) centre (25.6842, 9.585) ccw
  line L10 (24.4237, 16.8994) -> (30.5563, 9.766)
  line L11 (38.9174, 10.9962) -> (41.7768, 17.4348)
  line L12 (39.9427, 20.2466) -> (25.9341, 20.2032)
  arc A6 (30.5563, 9.766) -> (38.9174, 10.9962) centre (34.3478, 13.0255) ccw
  arc A7 (25.9341, 20.2032) -> (24.4237, 16.8994) centre (25.9403, 18.2032) ccw
  arc A8 (41.7768, 17.4348) -> (39.9427, 20.2466) centre (39.9489, 18.2466) ccw
  line L13 (39.6819, 7.6882) -> (40.0969, 8.6226)
  line L14 (40.9235, 10.4839) -> (44.5529, 18.6567)
  line L15 (47.3104, 20.4391) -> (66.1535, 20.3404)
  line L16 (68.9221, 18.4576) -> (72.2063, 10.2724)
  line L17 (70.3397, 7.5277) -> (42.7408, 7.6722)
  arc A9 (40.9235, 10.4839) -> (42.7408, 7.6722) centre (42.7513, 9.6722) ccw
  arc A10 (47.3104, 20.4391) -> (44.5529, 18.6567) centre (47.2947, 17.4391) ccw
  arc A11 (68.9221, 18.4576) -> (66.1535, 20.3404) centre (66.1378, 17.3404) ccw
  arc A12 (70.3397, 7.5277) -> (72.2063, 10.2724) centre (70.3501, 9.5277) ccw
  line L18 (71.6462, 18.4808) -> (74.5755, 10.555)
  line L19 (78.7729, 7.6151) -> (85.113, 7.5819)
  line L20 (88.9449, 9.6846) -> (93.7612, 17.3358)
  line L21 (92.0791, 20.4012) -> (73.061, 20.5008)
  arc A13 (73.061, 20.5008) -> (71.6462, 18.4808) centre (73.0532, 19.0008) ccw
  arc A14 (93.7612, 17.3358) -> (92.0791, 20.4012) centre (92.0686, 18.4012) ccw
  arc A15 (85.113, 7.5819) -> (88.9449, 9.6846) centre (85.1366, 12.0818) ccw
  arc A16 (74.5755, 10.555) -> (78.7729, 7.6151) centre (78.7965, 12.115) ccw
  line L22 (90.1988, 8.2439) -> (90.338, 8.4652)
  line L23 (91.1197, 9.7534) -> (96.4689, 18.5692)
  line L24 (99.9095, 20.4942) -> (116.4112, 20.4078)
  line L25 (119.3769, 17.0744) -> (118.6727, 10.7771)
  line L26 (115.6756, 8.1105) -> (91.9694, 8.2346)
  arc A17 (115.6756, 8.1105) -> (118.6727, 10.7771) centre (115.6913, 11.1105) ccw
  arc A18 (119.3769, 17.0744) -> (116.4112, 20.4078) centre (116.3955, 17.4078) ccw
  arc A19 (99.9095, 20.4942) -> (96.4689, 18.5692) centre (99.8886, 16.4942) ccw
  arc A20 (91.1197, 9.7534) -> (91.9694, 8.2346) centre (91.9746, 9.2346) ccw
  line L27 (121.0908, 17.6716) -> (120.4159, 10.4219)
  line L28 (122.3968, 8.2365) -> (132.5276, 8.1835)
  line L29 (136.1217, 10.3854) -> (138.1171, 14.3508)
  line L30 (133.8812, 20.8684) -> (123.9338, 20.3901)
  arc A21 (123.9338, 20.3901) -> (121.0908, 17.6716) centre (124.0779, 17.3935) ccw
  arc A22 (132.5276, 8.1835) -> (136.1217, 10.3854) centre (132.5486, 12.1834) ccw
  arc A23 (120.4159, 10.4219) -> (122.3968, 8.2365) centre (122.4073, 10.2365) ccw
  arc A24 (138.1171, 14.3508) -> (133.8812, 20.8684) centre (134.0974, 16.3736) ccw
  line L31 (146.332, 8.2412) -> (141.1164, 8.551)
  line L32 (140.3707, 12.9747) -> (141.4846, 13.4162)
  line L33 (143.741, 13.2057) -> (147.222, 11.0067)
  arc A25 (146.332, 8.2412) -> (147.222, 11.0067) centre (146.4209, 9.7386) ccw
  arc A26 (143.741, 13.2057) -> (141.4846, 13.4162) centre (142.4058, 11.0921) ccw
  arc A27 (140.3707, 12.9747) -> (138.9092, 11.8844) centre (141.6605, 9.721) ccw
  arc A28 (138.9092, 11.8844) -> (141.1164, 8.551) centre (141.2646, 11.0466) ccw
  line L34 (141.4284, 17.9658) -> (153.7485, 10.1717)
  line L35 (157.5534, 11.8877) -> (158.4978, 17.7645)
  line L36 (156.0426, 20.6611) -> (142.2381, 20.7334)
  arc A29 (142.2381, 20.7334) -> (141.4284, 17.9658) centre (142.2303, 19.2334) ccw
  arc A30 (158.4978, 17.7645) -> (156.0426, 20.6611) centre (156.0295, 18.1612) ccw
  arc A31 (153.7485, 10.1717) -> (157.5534, 11.8877) centre (155.085, 12.2844) ccw
  line L37 (159.7868, 17.1053) -> (158.8976, 11.2901)
  line L38 (161.3558, 8.4123) -> (172.1521, 8.3558)
  line L39 (175.3656, 9.9458) -> (182.6964, 19.6572)
  line L40 (181.9035, 21.2596) -> (164.7555, 21.3494)
  arc A32 (172.1521, 8.3558) -> (175.3656, 9.9458) centre (172.173, 12.3557) ccw
  arc A33 (182.6964, 19.6572) -> (181.9035, 21.2596) centre (181.8982, 20.2596) ccw
  arc A34 (164.7555, 21.3494) -> (159.7868, 17.1053) centre (164.7294, 16.3495) ccw
  arc A35 (158.8976, 11.2901) -> (161.3558, 8.4123) centre (161.3689, 10.9123) ccw
  line L41 (178.7313, 10.6243) -> (183.7183, 17.2309)
  line L42 (186.4137, 16.4005) -> (186.713, 10.2934)
  line L43 (184.7049, 8.1956) -> (179.9206, 8.2206)
  arc A36 (178.7313, 10.6243) -> (179.9206, 8.2206) centre (179.9285, 9.7206) ccw
  arc A37 (186.4137, 16.4005) -> (183.7183, 17.2309) centre (184.9155, 16.3271) ccw
  arc A38 (184.7049, 8.1956) -> (186.713, 10.2934) centre (184.7154, 10.1955) ccw
  line L44 (187.8816, 17.6171) -> (188.6139, 11.6076)
  line L45 (191.9985, 8.5321) -> (201.41, 8.2907)
  line L46 (203.2249, 11.2332) -> (199.0715, 18.9996)
  line L47 (196.0744, 20.8479) -> (190.9361, 20.979)
  arc A39 (190.9361, 20.979) -> (187.8816, 17.6171) centre (190.8596, 17.98) ccw
  arc A40 (199.0715, 18.9996) -> (196.0744, 20.8479) centre (195.9851, 17.3491) ccw
  arc A41 (188.6139, 11.6076) -> (191.9985, 8.5321) centre (192.0882, 12.0309) ccw
  arc A42 (201.41, 8.2907) -> (203.2249, 11.2332) centre (201.4613, 10.29) ccw
  line L48 (201.7255, 19.2137) -> (206.2094, 10.3318)
  line L49 (209.3021, 9.7195) -> (219.8405, 18.8208)
  line L50 (219.1921, 20.5776) -> (202.6234, 20.6644)
  arc A43 (219.8405, 18.8208) -> (219.1921, 20.5776) centre (219.1868, 19.5776) ccw
  arc A44 (202.6234, 20.6644) -> (201.7255, 19.2137) centre (202.6182, 19.6644) ccw
  arc A45 (206.2094, 10.3318) -> (209.3021, 9.7195) centre (207.9948, 11.2331) ccw
  line L51 (224.5057, 20.5679) -> (212.9932, 10.3357)
  line L52 (213.6523, 8.5883) -> (228.4256, 8.5109)
  line L53 (229.8322, 10.5527) -> (226.1025, 20.1816)
  arc A46 (212.9932, 10.3357) -> (213.6523, 8.5883) centre (213.6575, 9.5882) ccw
  arc A47 (226.1025, 20.1816) -> (224.5057, 20.5679) centre (225.17, 19.8204) ccw
  arc A48 (228.4256, 8.5109) -> (229.8322, 10.5527) centre (228.4335, 10.0109) ccw
  line L54 (229.0936, 17.8598) -> (231.3783, 11.5494)
  line L55 (235.5859, 8.5814) -> (240.2629, 8.5569)
  line L56 (242.0417, 11.4912) -> (238.0013, 19.1381)
  line L57 (235.1147, 20.9968) -> (231.5928, 21.2064)
  arc A49 (231.5928, 21.2064) -> (229.0936, 17.8598) centre (231.4443, 18.7108) ccw
  arc A50 (238.0013, 19.1381) -> (235.1147, 20.9968) centre (234.9067, 17.503) ccw
  arc A51 (231.3783, 11.5494) -> (235.5859, 8.5814) centre (235.6095, 13.0813) ccw
  arc A52 (240.2629, 8.5569) -> (242.0417, 11.4912) centre (240.2734, 10.5568) ccw
  line L58 (241.149, 18.3226) -> (242.9441, 15.1294)
  line L59 (244.7087, 15.1691) -> (246.705, 19.1272)
  line L60 (245.3658, 21.3027) -> (242.8924, 21.3027)
  arc A53 (242.8924, 21.3027) -> (241.149, 18.3226) centre (242.8924, 19.3027) ccw
  arc A54 (246.705, 19.1272) -> (245.3658, 21.3027) centre (245.3658, 19.8027) ccw
  arc A55 (242.9441, 15.1294) -> (244.7087, 15.1691) centre (243.8158, 15.6195) ccw
  line L61 (245.6044, 10.9717) -> (248.4424, 17.8482)
  line L62 (252.8821, 20.9374) -> (254.3603, 20.9913)
  line L63 (256.8976, 17.9771) -> (255.4793, 11.2514)
  line L64 (252.5282, 8.8705) -> (246.9831, 8.8995)
  arc A56 (252.5282, 8.8705) -> (255.4793, 11.2514) centre (252.5439, 11.8704) ccw
  arc A57 (256.8976, 17.9771) -> (254.3603, 20.9913) centre (254.4514, 18.493) ccw
  arc A58 (252.8821, 20.9374) -> (248.4424, 17.8482) centre (253.0643, 15.9408) ccw
  arc A59 (245.6044, 10.9717) -> (246.9831, 8.8995) centre (246.9909, 10.3995) ccw
  line L65 (258.6765, 18.9009) -> (259.7495, 18.0201)
  line L66 (260.4761, 17.7972) -> (268.7488, 18.5618)
  line L67 (268.76, 20.5522) -> (260.9859, 21.3597)
  line L68 (260.4799, 21.2804) -> (258.9084, 20.5892)
  arc A60 (268.7488, 18.5618) -> (268.76, 20.5522) centre (268.6567, 19.5576) ccw
  arc A61 (259.7495, 18.0201) -> (260.4761, 17.7972) centre (260.384, 18.793) ccw
  arc A62 (260.9859, 21.3597) -> (260.4799, 21.2804) centre (260.8825, 20.3651) ccw
  arc A63 (258.9084, 20.5892) -> (258.6765, 18.9009) centre (259.311, 19.6738) ccw
  line L69 (259.8934, 12.8272) -> (263.7712, 13.8599)
  line L70 (263.943, 15.7295) -> (263.2948, 16.0374)
  line L71 (260.2057, 16.3213) -> (260.5487, 16.4126)
  line L72 (258.7274, 14.4158) -> (258.6502, 13.9611)
  arc A64 (258.6502, 13.9611) -> (259.8934, 12.8272) centre (259.636, 13.7935) ccw
  arc A65 (260.5487, 16.4126) -> (258.7274, 14.4158) centre (261.1921, 13.9968) ccw
  arc A66 (263.2948, 16.0374) -> (260.2057, 16.3213) centre (261.3637, 11.9728) ccw
  arc A67 (263.7712, 13.8599) -> (263.943, 15.7295) centre (263.5138, 14.8262) ccw
  line L73 (260.859, 9.1138) -> (267.2715, 8.6455)
  line L74 (268.3665, 11.2722) -> (267.7988, 11.7671)
  line L75 (266.4949, 12.2596) -> (263.1929, 12.2769)
  line L76 (261.4041, 11.6969) -> (260.3408, 10.9178)
  arc A68 (260.3408, 10.9178) -> (260.859, 9.1138) centre (260.9318, 10.1112) ccw
  arc A69 (263.1929, 12.2769) -> (261.4041, 11.6969) centre (263.1771, 9.2769) ccw
  arc A70 (267.7988, 11.7671) -> (266.4949, 12.2596) centre (266.4845, 10.2596) ccw
  arc A71 (267.2715, 8.6455) -> (268.3665, 11.2722) centre (267.3808, 10.1415) ccw
  line L77 (292.8985, 19.3211) -> (296.229, 12.1883)
  line L78 (293.8125, 7.9342) -> (291.3456, 7.6849)
  line L79 (289.1444, 9.6747) -> (289.1444, 18.1058)
  arc A72 (291.5158, 20.6025) -> (289.1444, 18.1058) centre (291.6444, 18.1058) ccw
  arc A73 (292.8985, 19.3211) -> (291.5158, 20.6025) centre (290.6333, 18.2634) ccw
  arc A74 (293.8125, 7.9342) -> (296.229, 12.1883) centre (293.5108, 10.919) ccw
  arc A75 (289.1444, 9.6747) -> (291.3456, 7.6849) centre (291.1444, 9.6747) ccw
  line L80 (269.2858, 13.0247) -> (268.2548, 13.8227)
  line L81 (268.1983, 15.3572) -> (273.8556, 20.4432)
  line L82 (276.4233, 20.9179) -> (277.2957, 20.5828)
  line L83 (277.6094, 18.9089) -> (271.2123, 13.1004)
  line L84 (272.2544, 10.0762) -> (280.8351, 19.0578)
  line L85 (285.7475, 21.2208) -> (286.3302, 21.2332)
  line L86 (287.8621, 19.7335) -> (287.8621, 10.7978)
  line L87 (284.9291, 7.7985) -> (273.3725, 7.5404)
  arc A76 (285.7475, 21.2208) -> (280.8351, 19.0578) centre (285.8965, 14.2223) ccw
  arc A77 (287.8621, 19.7335) -> (286.3302, 21.2332) centre (286.3621, 19.7335) ccw
  arc A78 (284.9291, 7.7985) -> (287.8621, 10.7978) centre (284.8621, 10.7978) ccw
  arc A79 (272.2544, 10.0762) -> (273.3725, 7.5404) centre (273.339, 9.04) ccw
  arc A80 (277.6094, 18.9089) -> (277.2957, 20.5828) centre (276.9372, 19.6493) ccw
  arc A81 (276.4233, 20.9179) -> (273.8556, 20.4432) centre (275.527, 18.584) ccw
  arc A82 (268.1983, 15.3572) -> (268.2548, 13.8227) centre (268.8668, 14.6135) ccw
  arc A83 (269.2858, 13.0247) -> (271.2123, 13.1004) centre (270.2039, 14.2109) ccw
  line L88 (2.9636, 23.5975) -> (3.2504, 7.6166)
  line L89 (3.2504, 7.6166) -> (3.1633, 4.9975)
  dimension "d463" = 2.5
  dimension "d464" = 2
  dimension "d465" = 1.5
  dimension "d466" = 5
  dimension "d467" = 2
  dimension "d468" = 2
  dimension "d469" = 2
  dimension "d470" = 3
  dimension "d471" = 3
  dimension "d472" = 2
  dimension "d473" = 1.5
  dimension "d474" = 2
  dimension "d475" = 4.5
  dimension "d476" = 4.5
  dimension "d477" = 3
  dimension "d478" = 3
  dimension "d479" = 4
  dimension "d480" = 1
  dimension "d481" = 3
  dimension "d482" = 4
  dimension "d483" = 2
  dimension "d484" = 4.5
  dimension "d485" = 1.5
  dimension "d486" = 2.5
  dimension "d487" = 3.5
  dimension "d488" = 2.5
  dimension "d489" = 1.5
  dimension "d490" = 2.5
  dimension "d491" = 2.5
  dimension "d492" = 4
  dimension "d493" = 1
  dimension "d494" = 5
  dimension "d495" = 2.5
  dimension "d496" = 1.5
  dimension "d497" = 1.5
  dimension "d498" = 2
  dimension "d499" = 3
  dimension "d500" = 3.5
  dimension "d501" = 3.5
  dimension "d502" = 2
  dimension "d503" = 1
  dimension "d504" = 2
  dimension "d505" = 1
  dimension "d506" = 1
  dimension "d507" = 1.5
  dimension "d508" = 2.5
  dimension "d509" = 3.5
  dimension "d510" = 4.5
  dimension "d511" = 2
  dimension "d512" = 2
  dimension "d513" = 1.5
  dimension "d514" = 1
  dimension "d515" = 3
  dimension "d516" = 2.5
  dimension "d517" = 5
  dimension "d518" = 1.5
  dimension "d519" = 1
  dimension "d520" = 1
  dimension "d521" = 1
  dimension "d522" = 1
  dimension "d523" = 2.5
  dimension "d524" = 4.5
  dimension "d525" = 1
  dimension "d526" = 1
  dimension "d527" = 3
  dimension "d528" = 2
  dimension "d529" = 1.5
  dimension "d530" = 2.5
  dimension "d531" = 3
  dimension "d532" = 2
  dimension "d533" = 7
  dimension "d534" = 1.5
  dimension "d535" = 3
  dimension "d536" = 1.5
  dimension "d537" = 1
  dimension "d538" = 2.5
  dimension "d539" = 1
  dimension "d540" = 1.5
  constraint tangent L6 A0
  constraint tangent L4 A0
  constraint tangent L5 A1
  constraint tangent L6 A1
  constraint equal A0 A1
  constraint tangent L4 A2
  constraint tangent L5 A2
  constraint parallel L6 L7
  constraint perpendicular L6 L8
  constraint tangent L9 A3
  constraint tangent L7 A3
  constraint tangent L7 A4
  constraint tangent L8 A4
  constraint equal A3 A4
  constraint tangent L8 A5
  constraint tangent L9 A5
  constraint equal A3 A5
  constraint tangent L10 A6
  constraint tangent L11 A6
  constraint tangent L10 A7
  constraint tangent L12 A7
  constraint tangent L11 A8
  constraint tangent L12 A8
  constraint parallel L11 L13
  constraint parallel L11 L14
  constraint coincident L13.start L17
  constraint coincident L13.end L14
  constraint tangent L17 A9
  constraint tangent L14 A9
  constraint tangent L14 A10
  constraint tangent L15 A10
  constraint tangent L15 A11
  constraint tangent L16 A11
  constraint tangent L16 A12
  constraint tangent L17 A12
  constraint tangent L18 A13
  constraint tangent L21 A13
  constraint tangent L20 A14
  constraint tangent L21 A14
  constraint tangent L19 A15
  constraint tangent L20 A15
  constraint tangent L18 A16
  constraint tangent L19 A16
  constraint parallel L20 L22
  constraint tangent L25 A17
  constraint tangent L26 A17
  constraint tangent L24 A18
  constraint tangent L25 A18
  constraint tangent L23 A19
  constraint tangent L24 A19
  constraint coincident L22.start L26
  constraint coincident L22.end L23
  constraint tangent L26 A20
  constraint tangent L23 A20
  constraint tangent L27 A21
  constraint tangent L30 A21
  constraint tangent L28 A22
  constraint tangent L29 A22
  constraint tangent L28 A23
  constraint tangent L27 A23
  constraint tangent L30 A24
  constraint tangent L29 A24
  constraint tangent L31 A25
  constraint tangent L33 A25
  constraint tangent L32 A26
  constraint tangent L33 A26
  constraint tangent L32 A27
  constraint tangent L31 A28
  constraint coincident A27.end A28.start
  constraint tangent L34 A29
  constraint tangent L36 A29
  constraint tangent L35 A30
  constraint tangent L36 A30
  constraint tangent L34 A31
  constraint tangent L35 A31
  constraint tangent L38 A32
  constraint tangent L39 A32
  constraint tangent L39 A33
  constraint tangent L40 A33
  constraint tangent L37 A34
  constraint tangent L40 A34
  constraint tangent L37 A35
  constraint tangent L38 A35
  constraint parallel L39 L41
  constraint tangent L41 A36
  constraint tangent L43 A36
  constraint tangent L41 A37
  constraint tangent L42 A37
  constraint tangent L42 A38
  constraint tangent L43 A38
  constraint tangent L44 A39
  constraint tangent L47 A39
  constraint tangent L46 A40
  constraint tangent L47 A40
  constraint tangent L44 A41
  constraint tangent L45 A41
  constraint tangent L45 A42
  constraint tangent L46 A42
  constraint tangent L49 A43
  constraint tangent L50 A43
  constraint tangent L48 A44
  constraint tangent L50 A44
  constraint equal A43 A44
  constraint tangent L48 A45
  constraint tangent L49 A45
  constraint tangent L51 A46
  constraint tangent L52 A46
  constraint tangent L51 A47
  constraint tangent L53 A47
  constraint tangent L52 A48
  constraint tangent L53 A48
  constraint tangent L57 A49
  constraint tangent L54 A49
  constraint tangent L56 A50
  constraint tangent L57 A50
  constraint tangent L54 A51
  constraint tangent L55 A51
  constraint tangent L55 A52
  constraint tangent L56 A52
  constraint parallel L1 L60
  constraint tangent L58 A53
  constraint tangent L60 A53
  constraint tangent L59 A54
  constraint tangent L60 A54
  constraint tangent L58 A55
  constraint tangent L59 A55
  constraint tangent L63 A56
  constraint tangent L64 A56
  constraint tangent L62 A57
  constraint tangent L63 A57
  constraint tangent L61 A58
  constraint tangent L62 A58
  constraint tangent L61 A59
  constraint tangent L64 A59
  constraint tangent L66 A60
  constraint tangent L67 A60
  constraint tangent L65 A61
  constraint tangent L66 A61
  constraint tangent L67 A62
  constraint tangent L68 A62
  constraint equal A61 A62
  constraint tangent L68 A63
  constraint tangent L65 A63